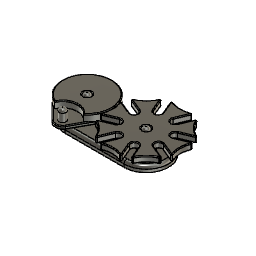
croix malte 8 branchesOK v2 (Autodesk Fusion 360 design; units mm, degrees)
Autodesk Fusion 360 part; units mm, degrees
sketch "Esquisse1" plane through (0, 0, 0) normal (0, 0, 1) x (1, 0, 0) in component "Component"
  line L0 (-80, -30) -> (0, -30)
  arc A0 (0, -30) -> (0, 30) centre (0, 0) ccw
  line L1 (0, 30) -> (-80, 30)
  arc A1 (-80, 30) -> (-80, -30) centre (-80, 0) ccw
  line L2 (-80, 0) -> (0, 0) construction
  point P0 (-40, 0)
  dimension "d1" = 80
  dimension "d2" = 60
  constraint tangent L0 A0
  constraint tangent A0 L1
  constraint parallel L0 L1
  constraint tangent L1 A1
  constraint tangent L0 A1
  constraint coincident A0.centre L2.end
  constraint horizontal L2
  constraint midpoint L2 P0
  measures "d1" distance of A0.end L1.end
  measures "d2" distance of L0 L1
extrude "Extrusion1" add sketch "Esquisse1" along normal blind 8 makes body 1 in component "Component"
sketch "Esquisse2" plane through (0, 0, 8) normal (0, 0, 1) x (-1, 0, 0) in component "Component"
  arc A0 (80, -30) -> (80, 30) centre (80, 0) ccw
  line L0 (80, 30) -> (0, 30)
  arc A1 (0, 30) -> (0, -30) centre (0, 0) ccw
  line L1 (0, -30) -> (80, -30)
  circle A2 centre (80, 0) radius 10
  dimension "d5" = 20
  constraint concentric A0 A2
  measures "d5" diameter of A2
extrude "Extrusion2" add sketch "Esquisse2" along normal blind 10 contours A2 bodies 1 in component "Component"
sketch "Esquisse3" plane through (0, 0, 18) normal (0, 0, 1) x (-1, 0, 0) in component "Component"
  circle A0 centre (80, 0) radius 10
  circle A1 centre (80, 0) radius 4.5
  dimension "d8" = 9
  constraint concentric A0 A1
  measures "d8" diameter of A1
extrude "Extrusion3" add sketch "Esquisse3" along normal blind 15 contours A1 bodies 1 in component "Component"
sketch "Esquisse4" plane through (0, 0, 8) normal (0, 0, 1) x (-1, 0, 0) in component "Component"
  circle A0 centre (80, 0) radius 10
  arc A1 (80, -30) -> (80, 30) centre (80, 0) ccw
  line L0 (80, 30) -> (0, 30)
  arc A2 (0, 30) -> (0, -30) centre (0, 0) ccw
  line L1 (0, -30) -> (80, -30)
  circle A3 centre (0, 0) radius 10
  dimension "d11" = 20
  constraint coincident A2.centre A3.centre
  measures "d11" diameter of A3
extrude "Extrusion4" add sketch "Esquisse4" along normal blind 15 contours A3 bodies 1 in component "Component"
sketch "Esquisse5" plane through (0, 0, 23) normal (0, 0, 1) x (-1, 0, 0) in component "Component"
  circle A0 centre (0, 0) radius 10
  circle A1 centre (0, 0) radius 4.5
  dimension "d14" = 9
  constraint coincident A0.centre A1.centre
  measures "d14" diameter of A1
extrude "Extrusion5" add sketch "Esquisse5" along normal blind 10 contours A1 bodies 1 in component "Component"
fillet "Congé1" radius 4 4 edges at (30, 0, 8) (-40, 30, 8) (-110, 0, 8) (-40, -30, 8) on bodies 1 in component "Component"
fillet "Congé2" radius 4 2 edges at (4.1955, 1.6273, 33) (-75.8045, 1.6273, 33) on bodies 1 in component "Component"
chamfer "Chanfrein1" distance 1 angle 45 2 edges at (-70.6767, 3.6162, 18) (9.3233, 3.6162, 23) on bodies 1 in component "Component"
sketch "Esquisse1 (2)" plane through (0, 0, 23) normal (0, 0, 1) x (-1, 0, 0) in component "Component'"
  circle A0 centre (0, 0) radius 4.5
  circle A1 centre (0, 0) radius 9
  circle A2 centre (0, 0) radius 5.25
  line L0 (0, 0) -> (-15.0917, -37.0338) construction
  line L1 (-14.1441, -47.9577) -> (-6.6911, -29.6687)
  arc A3 (-6.6911, -29.6687) -> (-15.9517, -25.8949) centre (-11.3214, -27.7818) ccw
  line L2 (-15.9517, -25.8949) -> (-23.4047, -44.1839)
  line L3 (7.0309, -29.59) -> (14.6932, -47.7924)
  arc A4 (16.2476, -25.7102) -> (7.0309, -29.59) centre (11.6393, -27.6501) ccw
  line L4 (23.9099, -43.9126) -> (16.2476, -25.7102)
  line L5 (25.8949, -15.9517) -> (44.1839, -23.4047)
  arc A5 (29.6687, -6.6911) -> (25.8949, -15.9517) centre (27.7818, -11.3214) ccw
  line L6 (47.9577, -14.1441) -> (29.6687, -6.6911)
  line L7 (29.59, 7.0309) -> (47.7924, 14.6932)
  arc A6 (25.7102, 16.2476) -> (29.59, 7.0309) centre (27.6501, 11.6393) ccw
  line L8 (43.9126, 23.9099) -> (25.7102, 16.2476)
  line L9 (15.9517, 25.8949) -> (23.4047, 44.1839)
  arc A7 (6.6911, 29.6687) -> (15.9517, 25.8949) centre (11.3214, 27.7818) ccw
  line L10 (14.1441, 47.9577) -> (6.6911, 29.6687)
  line L11 (-7.0309, 29.59) -> (-14.6932, 47.7924)
  arc A8 (-16.2476, 25.7102) -> (-7.0309, 29.59) centre (-11.6393, 27.6501) ccw
  line L12 (-23.9099, 43.9126) -> (-16.2476, 25.7102)
  line L13 (-25.8949, 15.9517) -> (-44.1839, 23.4047)
  arc A9 (-29.6687, 6.6911) -> (-25.8949, 15.9517) centre (-27.7818, 11.3214) ccw
  line L14 (-47.9577, 14.1441) -> (-29.6687, 6.6911)
  line L15 (-29.59, -7.0309) -> (-47.7924, -14.6932)
  arc A10 (-25.7102, -16.2476) -> (-29.59, -7.0309) centre (-27.6501, -11.6393) ccw
  line L16 (-43.9126, -23.9099) -> (-25.7102, -16.2476)
  arc A11 (48.4, 12.5475) -> (48.4, -12.5475) centre (80, 0) ccw
  arc A12 (47.9577, -14.1441) -> (48.4, -12.5475) centre (0, 0) ccw
  arc A13 (48.4, 12.5475) -> (47.7924, 14.6932) centre (0, 0) ccw
  arc A14 (25.3515, 43.0964) -> (43.0964, 25.3515) centre (56.5685, 56.5685) ccw
  arc A15 (-12.5475, 48.4) -> (12.5475, 48.4) centre (0, 80) ccw
  arc A16 (-43.0964, 25.3515) -> (-25.3515, 43.0964) centre (-56.5685, 56.5685) ccw
  arc A17 (-48.4, -12.5475) -> (-48.4, 12.5475) centre (-80, 0) ccw
  arc A18 (-25.3515, -43.0964) -> (-43.0964, -25.3515) centre (-56.5685, -56.5685) ccw
  arc A19 (12.5475, -48.4) -> (-12.5475, -48.4) centre (0, -80) ccw
  arc A20 (43.0964, -25.3515) -> (25.3515, -43.0964) centre (56.5685, -56.5685) ccw
  arc A21 (23.9099, -43.9126) -> (25.3515, -43.0964) centre (0, 0) ccw
  arc A22 (43.0964, -25.3515) -> (44.1839, -23.4047) centre (0, 0) ccw
  arc A23 (-14.1441, -47.9577) -> (-12.5475, -48.4) centre (0, 0) ccw
  arc A24 (12.5475, -48.4) -> (14.6932, -47.7924) centre (0, 0) ccw
  arc A25 (-43.9126, -23.9099) -> (-43.0964, -25.3515) centre (0, 0) ccw
  arc A26 (-25.3515, -43.0964) -> (-23.4047, -44.1839) centre (0, 0) ccw
  arc A27 (-47.9577, 14.1441) -> (-48.4, 12.5475) centre (0, 0) ccw
  arc A28 (-48.4, -12.5475) -> (-47.7924, -14.6932) centre (0, 0) ccw
  arc A29 (-23.9099, 43.9126) -> (-25.3515, 43.0964) centre (0, 0) ccw
  arc A30 (-43.0964, 25.3515) -> (-44.1839, 23.4047) centre (0, 0) ccw
  arc A31 (14.1441, 47.9577) -> (12.5475, 48.4) centre (0, 0) ccw
  arc A32 (-12.5475, 48.4) -> (-14.6932, 47.7924) centre (0, 0) ccw
  arc A33 (43.9126, 23.9099) -> (43.0964, 25.3515) centre (0, 0) ccw
  arc A34 (25.3515, 43.0964) -> (23.4047, 44.1839) centre (0, 0) ccw
  dimension "d22" = 10.5
  dimension "d23" = 100
  dimension "d24" = 10
  dimension "d25" = 30
  dimension "d27" = 360
  dimension "d28" = 68
  dimension "d30" = 360
  constraint coincident A0.centre A1.centre
  constraint concentric A2 A21
  constraint coincident L1.start A21
  constraint tangent L1 A3
  constraint tangent A3 L2
  constraint parallel L0 L2
  constraint coincident L0 A3.centre
  constraint concentric A21 A23
  constraint concentric A21 A25
  constraint concentric A21 A27
  constraint concentric A21 A29
  constraint concentric A21 A31
  constraint concentric A21 A33
  constraint concentric A12 A21
  constraint coincident A11.start A12
  constraint concentric A12 A13
  constraint concentric A21 A22
  constraint concentric A23 A24
  constraint concentric A25 A26
  constraint concentric A27 A28
  constraint concentric A29 A30
  constraint concentric A31 A32
  constraint concentric A33 A34
  measures "d22" diameter of A2
  measures "d23" diameter of A21
  measures "d24" distance of L1 L2
  measures "d25" distance of A0.centre A3.centre
  measures "d28" diameter of A11
extrude "Extrusion6" add sketch "Esquisse1 (2)" along normal blind 8 separate body contours A1 | L1 A3 L2 L3 A4 L4 L5 A5 L6 L7 A6 L8 L9 A7 L10 L11 A8 L12 L13 A9 L14 L15 A10 L16 A11 A12 A13 A14 A15 A16 A17 A18 A19 A20 A21 A22 A23 A24 A25 A26 A27 A28 A29 A30 A31 A32 A33 A34 makes body 2 in component "Component"
chamfer "Chanfrein2" distance 1 angle 45 2 edges at (3.5671, -3.852, 31) (4.1955, -1.6273, 23) on bodies 1 2 in component "Component"
fillet "Congé3" radius 1 3 edges at (-10.4176, -38.8132, 23) (-9.4345, -23.1515, 23) (-19.6782, -35.0394, 23) 48 faces at (7.5095, -24.8314, 25.6667) (21.3558, -37.8452, 28.3333) (9.585, -35.6574, 25.6667) (25.1927, -43.1894, 28.3333) (40.5249, -26.5919, 28.3333) (44.0674, -23.6234, 28.3333) (41.8614, -11.6598, 28.3333) (25.6664, -15.8519, 28.3333) (31.9912, -18.436, 25.6667) (48.0095, -13.9674, 25.6667) (46.7469, -7.0873, 25.6667) (37.8452, 21.3558, 25.6667) (29.3579, 6.9399, 28.3333) (35.6574, 9.585, 25.6667) (47.8646, 14.4561, 28.3333) (43.4651, 24.7141, 28.3333) (31.5387, 33.5575, 25.6667) (23.6234, 44.0674, 28.3333) (18.436, 31.9912, 28.3333) (6.3217, 27.7219, 28.3333) (11.6598, 41.8614, 25.6667) (13.9674, 48.0095, 25.6667) (11.2097, 47.9011, 25.6667) (-14.4561, 47.8646, 28.3333) (-21.3558, 37.8452, 25.6667) (-6.9399, 29.3579, 28.3333) (-9.585, 35.6574, 28.3333) (-24.5539, 43.5558, 28.3333) (-36.8852, 28.8455, 25.6667) (-44.0674, 23.6234, 28.3333) (-31.9912, 18.436, 25.6667) (-24.425, 15.0271, 28.3333) (-41.8614, 11.6598, 25.6667) (-48.3535, 12.7256, 28.3333) (-46.1199, 2.8525, 28.3333) (-47.8646, -14.4561, 28.3333) (-35.6574, -9.585, 25.6667) (-27.8968, -6.6453, 28.3333) (-37.8452, -21.3558, 28.3333) (-43.8243, -24.0714, 25.6667) (-34.6287, -30.5947, 25.6667) (-24.2759, -43.7113, 28.3333) (-18.436, -31.9912, 25.6667) (-6.3217, -27.7219, 28.3333) (-11.6598, -41.8614, 28.3333) (-12.7256, -48.3535, 28.3333) (1.4275, -46.03, 25.6667) (12.7872, -48.3372, 28.3333) on bodies 2 in component "Component"
sketch "Esquisse1 (3)" plane through (0, 0, 18) normal (0, 0, 1) x (-1, 0, 0) in component "Component''"
  circle A0 centre (80, 0) radius 4.5
  circle A1 centre (80, 0) radius 9
  circle A2 centre (80, 0) radius 5.25
  circle A3 centre (80, 0) radius 33.5
  line L0 (80, 0) -> (80, 55) construction
  line L1 (106.7354, 20.1859) -> (87.9807, 45.0256)
  arc A4 (87.9807, 45.0256) -> (72.0193, 45.0256) centre (80, 39) ccw
  line L2 (72.0193, 45.0256) -> (53.2646, 20.1859)
  dimension "d39" = 10.5
  dimension "d40" = 67
  dimension "d41" = 39
  dimension "d42" = 10
  constraint concentric A0 A2
  constraint concentric A2 A3
  constraint coincident A0.centre A1.centre
  constraint vertical L0
  constraint coincident A3 L1.start
  constraint tangent L1 A4
  constraint coincident A3 L2.end
  constraint tangent A3 L2
  constraint tangent A3 L1
  constraint tangent A4 L2
  constraint coincident L0 A4.centre
  measures "d39" diameter of A2
  measures "d40" diameter of A3
  measures "d41" distance of A0.centre A4.centre
  measures "d42" radius of A4
extrude "Extrusion1'" add sketch "Esquisse1 (3)" along normal blind 4.5 separate body contours A1 | A3 | A3 L1 A4 L2 makes body 3 in component "Component''"
sketch "Esquisse2 (2)" plane through (0, 0, 22.5) normal (0, 0, 1) x (-1, 0, 0) in component "Component''"
  circle A0 centre (80, 0) radius 5.25
  line L0 (72.0193, 45.0256) -> (53.2646, 20.1859)
  arc A1 (53.2646, 20.1859) -> (106.7354, 20.1859) centre (80, 0) ccw
  line L1 (106.7354, 20.1859) -> (87.9807, 45.0256)
  arc A2 (87.9807, 45.0256) -> (72.0193, 45.0256) centre (80, 39) ccw
  circle A3 centre (80, 0) radius 5.25
  arc A4 (62.8205, 28.7596) -> (97.1795, 28.7596) centre (80, 0) ccw
  arc A5 (62.8205, 28.7596) -> (97.1795, 28.7596) centre (80, 39) ccw
  dimension "d45" = 10.5
  dimension "d46" = 67
  dimension "d47" = 40
  constraint concentric A0 A3
  constraint concentric A3 A4
  constraint concentric A2 A5
  measures "d45" diameter of A3
  measures "d46" diameter of A4
  measures "d47" diameter of A5
extrude "Extrusion2'" add sketch "Esquisse2 (2)" along normal blind 8.5 contours A1 A4 A5 bodies 3 in component "Component''"
sketch "Esquisse3 (2)" plane through (0, 0, 22.5) normal (0, 0, 1) x (-1, 0, 0) in component "Component''"
  arc A0 (106.7354, 20.1859) -> (97.1795, 28.7596) centre (80, 0) ccw
  line L0 (106.7354, 20.1859) -> (87.9807, 45.0256)
  arc A1 (87.9807, 45.0256) -> (72.0193, 45.0256) centre (80, 39) ccw
  line L1 (72.0193, 45.0256) -> (53.2646, 20.1859)
  arc A2 (62.8205, 28.7596) -> (53.2646, 20.1859) centre (80, 0) ccw
  arc A3 (62.8205, 28.7596) -> (97.1795, 28.7596) centre (80, 39) ccw
  circle A4 centre (80, 39) radius 4.5
  dimension "d50" = 9
  constraint concentric A1 A4
  measures "d50" diameter of A4
extrude "Extrusion3'" add sketch "Esquisse3 (2)" along normal blind 15 contours A4 bodies 3 in component "Component''"
chamfer "Chanfrein1'" distance 1 angle 45 2 edges at (-75.1053, -1.8985, 18) (-75.1053, -1.8985, 31) on bodies 3 in component "Component''"
fillet "Congé1'" radius 1 9 edges at (-80, 33.5, 31) (-97.358, -32.6058, 22.5) (-80, -49, 22.5) (-62.642, -32.6058, 22.5) (-62.642, -32.6058, 18) (-80, 33.5, 18) (-97.358, -32.6058, 18) (-80, -49, 18) (-80, -19, 31) on bodies 3 in component "Component''"
fillet "Congé2'" radius 4 1 edges at (-75.8045, -37.3727, 37.5) on bodies 3 in component "Component''"
copy_body "CutPasteBodies1" bodies 2 removing the originals makes body 4 in component "Component'"
component "Component" placed x (1, 0, 0) y (0, 1, 0) z (0, 0, 1) at (0, 0, 0)
component "Component'" placed x (0.705733, -0.708478, 0) y (0.708478, 0.705733, 0) z (0, 0, 1) at (0, 0, 0)
component "Component''" placed x (0.990258, 0.139244, 0) y (-0.139244, 0.990258, 0) z (0, 0, 1) at (-0.7793, 11.1395, 0)
